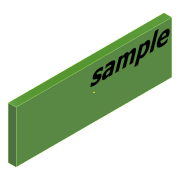
# Autodesk Inventor part: sample
Saved by Autodesk Inventor 2021 (Build 250183000, 183)
## iProperties
Created: 2022-02-10
Part Number: sample
Material: Типовые
Document SubType Name: Modeling
Designer: Тиннелла о Каллинике
Density: 1 g/cm^3
Appearance: Зеленовато-желтый
Author: Тиннелла о Каллинике
Autodesk Inventor part; units mm, degrees
ref_plane "YZ Plane" through (0, 0, 0) normal (1, 0, 0) x (0, 1, 0)
ref_plane "XZ Plane" through (0, 0, 0) normal (0, 1, 0) x (-1, 0, 0)
ref_plane "XY Plane" through (0, 0, 0) normal (0, 0, 1) x (1, 0, 0)
sketch "Эскиз1" plane through (0, 0, 0) normal (1, 0, 0) x (0, 1, 0)
  line L0 (5, 15) -> (-5, 15)
  line L1 (-5, 15) -> (-5, -15)
  line L2 (-5, -15) -> (5, -15)
  line L3 (5, -15) -> (5, 15)
  point P0 (0, 0)
  point P1 (5, 0)
  point P2 (0, -15)
  dimension "d0" = 30
  dimension "d1" = 10
  constraints: 8 end point, 2 midpoint, 2 parallel, 1 horizontal, 1 horizontal alignment, 1 perpendicular, 1 vertical alignment
  measures "d0" distance of L2.end L0.start
  measures "d1" distance of L1.end L2.end
extrude "Выдавливание1" add sketch "Эскиз1" along normal blind 1.5
sketch "Эскиз2" plane through (1.5, 0, 0) normal (1, 0, 0) x (0, 0, -1)
  line L0 (-0.885, 4.33) -> (22.1239, 4.33) construction
  line L1 (22.1239, 4.33) -> (22.1239, 2.5601) construction
  line L2 (22.1239, 2.5601) -> (-0.885, 2.5601) construction
  line L3 (-0.885, 2.5601) -> (-0.885, 4.33) construction
  point P0 (0, 0)
  constraints: 2 other
